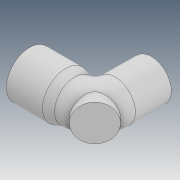
# Autodesk Inventor part: MtoF90Degree
Saved by Autodesk Inventor 2020 (Build 240168000, 168)
## iProperties
Created: 2020-05-04
Part Number: MtoF90Degree
Material: Generic
Document SubType Name: Modeling
Designer: Theo Cominotto
Density: 1 g/cm^3
Appearance: Default
Author: Theo Cominotto
Autodesk Inventor part; units mm, degrees
ref_plane "XZ Plane" through (0, 0, 0) normal (0, 1, 0) x (-1, 0, 0)
ref_plane "XY Plane" through (0, 0, 0) normal (0, 0, 1) x (1, 0, 0)
sketch "Sketch1" plane through (0, 0, 0) normal (0, 0, 1) x (1, 0, 0)
  line L0 (0, 0) -> (0, 11.2) construction
  line L1 (0, 0) -> (20, 0) construction
  line L2 (20, 0) -> (20, 11) construction
  line L3 (0, 11.2) -> (0, 12.8)
  line L4 (0, 11.2) -> (20, 11)
  line L5 (0, 12.8) -> (20, 12.8)
  line L6 (0, 12.8) -> (20, 12.8) construction
  line L7 (20, 12.8) -> (20, 11)
  line L8 (20, 0) -> (25, 0) construction
  line L9 (25, 0) -> (25, 11.2) construction
  line L10 (25, 11.2) -> (20, 12.8)
  line L11 (25, 11.2) -> (25, 9.4)
  line L12 (25, 9.4) -> (20, 11)
  dimension "d0" = 11.2
  dimension "d1" = 20
  dimension "d2" = 11
  dimension "d3" = 1.6
  dimension "d4" = 0
  dimension "d5" = 5
  dimension "d6" = 11.2
  dimension "d7" = 1.8
  constraints: 26 end point, 3 horizontal, 3 perpendicular, 2 vertical, 1 collinear, 1 point on line
  measures "d0" distance of L0.start L0.end
  measures "d1" distance of L0.start L1.end
  measures "d2" distance of L1.end L2.end
  measures "d3" distance of L0.end L3.end
  measures "d4" distance between parallel lines of L5 L6
  measures "d5" distance of L1.end L8.end
  measures "d6" distance of L8.end L9.end
  measures "d7" distance of L9.end L11.end
revolve "Revolution1" add sketch "Sketch1" angle 360 about axis through (0, 0, 0) along (1, 0, 0)
sketch "Sketch2" plane through (25, 0, 0) normal (1, 0, 0) x (0, 0, -1)
  line L0 (0, 0) -> (11.2, 0) construction
  circle A0 centre (0, 0) radius 9.4 projected
  circle A1 centre (0, 0) radius 11.2 projected
  line L1 (11.2, 0) -> (11.2, 12.8) construction
  dimension "d9" = 11.2
  constraints: 4 end point, 1 horizontal, 1 horizontal alignment, 1 vertical
  measures "d9" distance of L0.start L0.end
revolve "Revolution2" add sketch "Sketch2" angle 90 about axis through (25, 0, -11.2) along (0, 1, 0)
sketch "Sketch3" plane through (0, 0, 0) normal (0, 1, 0) x (-1, 0, 0)
  line L0 (-47.4, -11.2) -> (-25, -11.2) construction
  line L1 (-36.2, -11.2) -> (-36.2, -31.2) construction
  line L2 (-36.2, -31.2) -> (-25.2, -31.2) construction
  line L3 (-25.2, -31.2) -> (-25, -11.2)
  line L4 (-25, -11.2) -> (-26.8, -11.2)
  arc A0 (-25, -9.4) -> (-26.8, -11.2) centre (-25, -11.2) ccw projected
  line L5 (-26.8, -11.2) -> (-26.8, -31.2)
  line L6 (-25.2, -31.2) -> (-26.8, -31.2)
  point P0 (0, 0)
  dimension "d11" = 20
  dimension "d12" = 11
  constraints: 12 end point, 4 perpendicular, 2 point on line, 1 midpoint, 1 point on circle
  measures "d11" distance of L1.start L1.end
  measures "d12" distance of L1.end L2.end
revolve "Revolution3" add sketch "Sketch3" angle 360 about axis through (36.2, 0, -11.2) along (0, 0, -1)
ref_plane "Work Plane2" through (23.3345, 0, 23.3345) normal (0.7071, 0, 0.7071) x (0, 1, 0)
ref_plane "Work Plane1" through (0, 0, 0) normal (0.7071, 0, 0.7071) x (0, 1, 0)
sketch "Sketch4" plane through (23.3345, 0, 23.3345) normal (0.7071, 0, 0.7071) x (0, 1, 0)
  ellipse E0 centre (0, -17.6777) end of major axis (11.2, -17.6777) minor radius 7.9196 construction
  ellipse E1 centre (0, -33.5169) end of major axis (11.2, -33.5169) minor radius 7.9196 construction
  line L0 (0, -17.6777) -> (0, -33.5169) construction
  circle A0 centre (0, -25.5973) radius 10
  point P0 (0, 0)
  dimension "d16" = 20
  constraints: 2 end point, 2 vertical alignment, 1 centre point, 1 coincident, 1 vertical
  measures "d16" diameter of A0
extrude "Extrusion1" add sketch "Sketch4" against normal up to surface
equation "\"d0\" = 0.5 * TMEnd"
equation "\"d1\" = TDepth"
equation "\"d2\" = 0.5 * TMStart"
equation "\"d3\" = WallT"
equation "\"d6\" = 0.5 * TMEnd"
equation "\"d7\" = WallT + 0.5 * TMEnd - 0.5 * TMStart"
equation "\"d9\" = BendR"
equation "\"d11\" = TDepth"
equation "\"d12\" = 0.5 * TMStart"
equation "\"TMEnd\" = 22.4"
equation "\"TDepth\" = 20"
equation "\"TMStart\" = 22"
equation "\"WallT\" = 1.6"
equation "\"BendR\" = 11.2"
body "Solid1"
